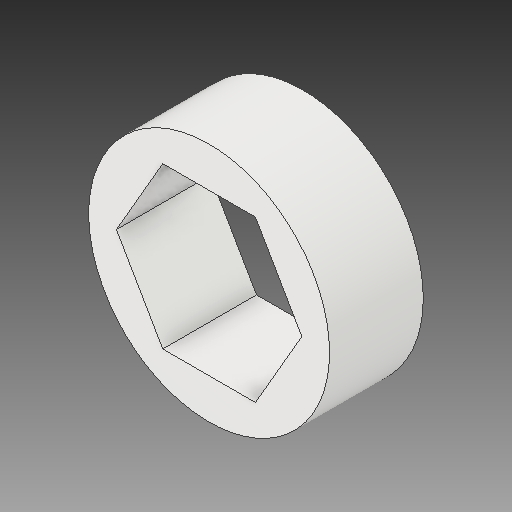
# Autodesk Inventor part: ARM_018_0.5inHexSpacer
Saved by Autodesk Inventor 2018.3 (Build 223284000, 284)
## iProperties
Created: 2020-02-02
Part Number: ARM_018_0.5inHexSpacer
Material: ABS Plastic
Document SubType Name: Modeling
Designer: 22barlalex
Density: 1.06 g/cm^3
Appearance: Smooth - White
Mass: 1.14265 g
Surface Area: 10.6085 cm^2
Volume: 1.07797 cm^3
Author: 22barlalex
Autodesk Inventor part; units mm, degrees
ref_plane "YZ Plane" through (0, 0, 0) normal (1, 0, 0) x (0, 1, 0)
ref_plane "XZ Plane" through (0, 0, 0) normal (0, 1, 0) x (-1, 0, 0)
ref_plane "XY Plane" through (0, 0, 0) normal (0, 0, 1) x (1, 0, 0)
sketch "Sketch1" plane through (0, 0, 0) normal (0, 0, 1) x (1, 0, 0)
  circle A0 centre (0, 0) radius 9.525
  line L0 (3.6662, 6.35) -> (7.3323, 0)
  line L1 (7.3323, 0) -> (3.6662, -6.35)
  line L2 (3.6662, -6.35) -> (-3.6662, -6.35)
  line L3 (-3.6662, -6.35) -> (-7.3323, 0)
  line L4 (-7.3323, 0) -> (-3.6662, 6.35)
  line L5 (-3.6662, 6.35) -> (3.6662, 6.35)
  dimension "d0" = 19.05
  dimension "d1" = 12.7
  constraints: 12 end point, 2 coincident, 1 centre point, 1 horizontal alignment, 13 other
  measures "d0" diameter of A0
  measures "d1" distance between parallel lines of L5 L2
extrude "Extrusion1" add sketch "Sketch1" along normal blind 7.4168
body "Solid1"
